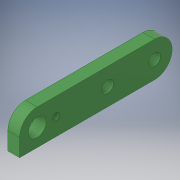
# Autodesk Inventor part: Cross Brace Plate
Saved by Autodesk Inventor 2017 (Build 210142000, 142)
## iProperties
Created: 2017-01-12
Part Number: Cross Brace Plate
Material: Generic
Document SubType Name: Modeling
Designer: Ben
Density: 1 g/cm^3
Appearance: Smooth - Dark Forest Green
Author: Ben
Autodesk Inventor part; units mm, degrees
ref_plane "YZ Plane" through (0, 0, 0) normal (1, 0, 0) x (0, 1, 0)
ref_plane "XZ Plane" through (0, 0, 0) normal (0, 1, 0) x (-1, 0, 0)
ref_plane "XY Plane" through (0, 0, 0) normal (0, 0, 1) x (1, 0, 0)
sketch "Sketch1" plane through (0, 0, 0) normal (1, 0, 0) x (0, 1, 0)
  circle A0 centre (0, 0) radius 4.7625
  line L0 (-9.525, 9.525) -> (-9.525, -63.5)
  line L1 (9.525, -63.5) -> (9.525, 0)
  line L2 (0, 9.525) -> (-9.525, 9.525)
  arc A1 (9.525, 0) -> (0, 9.525) centre (0, 0) ccw
  circle A2 centre (0, -38.1) radius 3.175
  circle A3 centre (0, -63.5) radius 3.175
  line L3 (0, -63.5) -> (0, 0) construction
  arc A4 (-9.525, -63.5) -> (9.525, -63.5) centre (0, -63.5) ccw
  circle A5 centre (0, -10.16) radius 1.905
  dimension "d0" = 9.525
  dimension "d3" = 19.05
  dimension "d4" = 9.525
  dimension "d5" = 9.525
  dimension "d6" = 9.525
  dimension "d7" = 6.35
  dimension "d9" = 25.4
  dimension "d10" = 38.1
  dimension "d13" = 3.81
  dimension "d14" = 10.16
  constraints: 8 end point, 6 centre point, 4 point on circle, 3 tangent, 2 coincident, 2 point on line, 2 vertical, 1 equal radius, 1 perpendicular
  measures "d0" diameter of A0
  measures "d3" distance between parallel lines of L0 L1
  measures "d4" distance from line of L0 point (0, 0)
  measures "d5" distance from line of L2 point (0, 0)
  measures "d6" radius of A1
  measures "d7" diameter of A2
  measures "d9" distance of A2.centre L3.start
  measures "d10" distance of point (0, 0) A2.centre
  measures "d13" diameter of A5
  measures "d14" distance of point (0, 0) A5.centre
extrude "Extrusion1" add sketch "Sketch1" along normal blind 6.35
equation "\"d4\" = 0.5 * d3"
equation "\"d5\" = d4"
equation "\"d6\" = d4"
body "Solid1"
